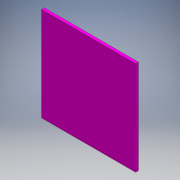
# Autodesk Inventor part: plaque
Saved by Autodesk Inventor 2017 (Build 210142000, 142)
## iProperties
Created: 2017-04-16
Part Number: plaque
Material: Generic
Document SubType Name: Modeling
Designer: franc
Density: 1 g/cm^3
Appearance: Default
Author: franc
Autodesk Inventor part; units mm, degrees
ref_plane "YZ Plane" through (0, 0, 0) normal (1, 0, 0) x (0, 1, 0)
ref_plane "XZ Plane" through (0, 0, 0) normal (0, 1, 0) x (-1, 0, 0)
ref_plane "XY Plane" through (0, 0, 0) normal (0, 0, 1) x (1, 0, 0)
sketch "Sketch1" plane through (0, 0, 0) normal (0, 1, 0) x (-1, 0, 0)
  line L0 (34, 64.6479) -> (-136, 64.6479)
  line L1 (-136, 64.6479) -> (-136, -105.3521)
  line L2 (-136, -105.3521) -> (34, -105.3521)
  line L3 (34, -105.3521) -> (34, 64.6479)
  circle A0 centre (31, 61.6479) radius 1
  circle A1 centre (15, 61.6479) radius 1
  circle A2 centre (31, 45.6479) radius 1
  circle A3 centre (15, 45.6479) radius 1
  point P0 (0, 0)
  dimension "d0" = 170
  dimension "d1" = 170
  dimension "d4" = 3
  dimension "d5" = 3
  dimension "d6" = 2
  dimension "d7" = 16
  dimension "d8" = 3
  dimension "d9" = 2
  dimension "d10" = 2
  dimension "d11" = 3
  dimension "d12" = 16
  dimension "d13" = 16
  dimension "d14" = 16
  dimension "d15" = 2
  constraints: 8 end point, 4 centre point, 2 parallel, 1 horizontal, 1 perpendicular
  measures "d0" distance of L2.end L0.start
  measures "d1" distance of L0.start L0.end
  measures "d4" distance from line of L0 A0.centre
  measures "d5" distance from line of A0.centre L3
  measures "d6" diameter of A0
  measures "d7" distance of A1.centre A0.centre
  measures "d8" distance from line of L0 A1.centre
  measures "d9" diameter of A1
  measures "d10" diameter of A2
  measures "d11" distance from line of L3 A2.centre
  measures "d12" distance of A0.centre A2.centre
  measures "d13" distance of A1.centre A3.centre
  measures "d14" distance of A2.centre A3.centre
  measures "d15" diameter of A3
extrude "Extrusion1" add sketch "Sketch1" along normal blind 5
body "Solid1"
